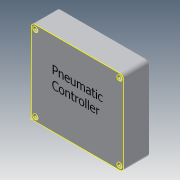
# Autodesk Inventor part: Pneumatic controller
Saved by Autodesk Inventor 2014 (Build 180170000, 170)
## iProperties
Created: 2016-01-12
Part Number: Pneumatic controller
Material: Generic
Document SubType Name: Modeling
Designer: Paul
Density: 1 g/cm^3
Appearance: Default
Author: Paul
Autodesk Inventor part; units mm, degrees
ref_plane "YZ Plane" through (0, 0, 0) normal (1, 0, 0) x (0, 1, 0)
ref_plane "XZ Plane" through (0, 0, 0) normal (0, 1, 0) x (-1, 0, 0)
ref_plane "XY Plane" through (0, 0, 0) normal (0, 0, 1) x (1, 0, 0)
sketch "Sketch1" plane through (0, 0, 0) normal (0, 0, 1) x (1, 0, 0)
  line L0 (0, 0) -> (69.85, 0)
  line L1 (69.85, 0) -> (69.85, 63.5)
  line L2 (69.85, 63.5) -> (0, 63.5)
  line L3 (0, 63.5) -> (0, 0)
  dimension "d0" = 69.85
  dimension "d1" = 63.5
  constraints: 8 end point, 2 parallel, 1 horizontal, 1 perpendicular
  measures "d0" distance of L2.end L1.end
  measures "d1" distance of L1.end L0.end
extrude "Extrusion1" add sketch "Sketch1" along normal blind 19.05
fillet "Fillet1" radius 3.175 4 edges at (0, 0, 9.525) (69.85, 63.5, 9.525) (69.85, 0, 9.525) (0, 63.5, 9.525)
sketch "Sketch2" plane through (0, 0, 19.05) normal (0, 0, 1) x (1, 0, 0)
  arc A0 (3.175, 63.5) -> (0, 60.325) centre (3.175, 60.325) ccw projected
  arc A1 (0, 3.175) -> (3.175, 0) centre (3.175, 3.175) ccw projected
  arc A2 (66.675, 0) -> (69.85, 3.175) centre (66.675, 3.175) ccw projected
  arc A3 (69.85, 60.325) -> (66.675, 63.5) centre (66.675, 60.325) ccw projected
  line L0 (11.6147, 49.5529) -> (59.516, 49.5529) construction
  line L1 (59.516, 49.5529) -> (59.516, 14.9717) construction
  line L2 (59.516, 14.9717) -> (11.6147, 14.9717) construction
  line L3 (11.6147, 14.9717) -> (11.6147, 49.5529) construction
  point P0 (0, 0)
  constraints: 2 other
hole "Hole1" at (3.175, 60.325, 19.05) at (66.675, 60.325, 19.05) at (3.175, 3.175, 19.05) at (66.675, 3.175, 19.05) direction (0, 0, -1) diameter 3.9624 depth 25.4 tip angle 118
sketch "Sketch3" plane through (0, 0, 19.05) normal (0, 0, 1) x (1, 0, 0)
  circle A0 centre (3.175, 3.175) radius 1.9812 projected
  circle A1 centre (3.175, 60.325) radius 1.9812 projected
  circle A2 centre (66.675, 60.325) radius 1.9812 projected
  circle A3 centre (66.675, 3.175) radius 1.9812 projected
  arc A4 (3.175, 63.5) -> (0, 60.325) centre (3.175, 60.325) ccw projected
  line L0 (0, 60.325) -> (0, 3.175) projected
  arc A5 (0, 3.175) -> (3.175, 0) centre (3.175, 3.175) ccw projected
  line L1 (3.175, 0) -> (66.675, 0) projected
  arc A6 (66.675, 0) -> (69.85, 3.175) centre (66.675, 3.175) ccw projected
  line L2 (69.85, 3.175) -> (69.85, 60.325) projected
  arc A7 (69.85, 60.325) -> (66.675, 63.5) centre (66.675, 60.325) ccw projected
  line L3 (66.675, 63.5) -> (3.175, 63.5) projected
  line L4 (15.7133, 43.9174) -> (63.8707, 43.9174) construction
  line L5 (63.8707, 43.9174) -> (63.8707, 14.9717) construction
  line L6 (63.8707, 14.9717) -> (15.7133, 14.9717) construction
  line L7 (15.7133, 14.9717) -> (15.7133, 43.9174) construction
  point P0 (0, 0)
  constraints: 2 other
body "Solid1"
